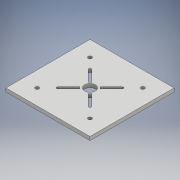
# Autodesk Inventor part: Base Robot
Saved by Autodesk Inventor 2017 (Build 210142000, 142)
## iProperties
Created: 2021-03-08
Part Number: Base Robot
Material: Generic
Document SubType Name: Modeling
Designer: Lenovo Y900
Density: 1 g/cm^3
Appearance: Default
Author: Lenovo Y900
Autodesk Inventor part; units mm, degrees
ref_plane "YZ Plane" through (0, 0, 0) normal (1, 0, 0) x (0, 1, 0)
ref_plane "XZ Plane" through (0, 0, 0) normal (0, 1, 0) x (-1, 0, 0)
ref_plane "XY Plane" through (0, 0, 0) normal (0, 0, 1) x (1, 0, 0)
sketch "Sketch1" plane through (0, 0, 0) normal (0, 0, 1) x (1, 0, 0)
  circle A0 centre (-22, 22) radius 1.5
  circle A1 centre (22, 22) radius 1.5
  circle A2 centre (22, -22) radius 1.5
  circle A3 centre (-22, -22) radius 1.5
  circle A4 centre (0, 0) radius 4.5
  line L0 (14.8492, 13.435) -> (-14.8492, -13.435) construction
  line L1 (13.435, -14.8492) -> (-13.435, 14.8492) construction
  line L2 (-14.8492, 13.435) -> (14.8492, -13.435) construction
  line L3 (-12.7279, 14.1421) -> (-3.4762, 4.8904) construction
  line L4 (-4.8904, 3.4762) -> (-14.1421, 12.7279)
  line L5 (-4.8904, -3.4762) -> (-14.1421, -12.7279)
  line L6 (-12.7279, -14.1421) -> (-3.4762, -4.8904)
  line L7 (12.7279, -14.1421) -> (3.4762, -4.8904)
  line L8 (-0.6718, -0.7425) -> (-0.7425, -0.6718)
  line L9 (0.6718, 0.7425) -> (0.7071, 0.7071)
  line L10 (4.8904, -3.4762) -> (14.1421, -12.7279)
  line L11 (0.6718, -0.7425) -> (0.7425, -0.6718)
  line L12 (4.8904, 3.4762) -> (14.1421, 12.7279)
  line L13 (12.7279, 14.1421) -> (3.4762, 4.8904)
  line L14 (-0.6718, 0.7425) -> (-0.7425, 0.6718)
  arc A5 (-12.7279, 14.1421) -> (-14.1421, 12.7279) centre (-13.435, 13.435) ccw
  arc A6 (14.1421, 12.7279) -> (12.7279, 14.1421) centre (13.435, 13.435) ccw
  arc A7 (-14.1421, -12.7279) -> (-12.7279, -14.1421) centre (-13.435, -13.435) ccw
  arc A8 (12.7279, -14.1421) -> (14.1421, -12.7279) centre (13.435, -13.435) ccw
  line L15 (-20.9393, -20.9393) -> (-22, -22)
  line L16 (-22, 22) -> (-20.9393, 20.9393)
  line L17 (22, 22) -> (20.9393, 20.9393)
  line L18 (20.9393, -20.9393) -> (22, -22)
  line L19 (-13.435, -14.8492) -> (4.0255, 4.4492) construction
  line L20 (12.9433, 14.3058) -> (13.435, 14.8492) construction
  line L21 (-12.7279, 14.1421) -> (-3.4762, 4.8904)
  arc A9 (-3.4762, 4.8904) -> (-4.8904, 3.4762) centre (0, 0) ccw
  arc A10 (-4.8904, -3.4762) -> (-3.4762, -4.8904) centre (0, 0) ccw
  arc A11 (3.4762, -4.8904) -> (4.8904, -3.4762) centre (0, 0) ccw
  arc A12 (4.8904, 3.4762) -> (3.4762, 4.8904) centre (0, 0) ccw
  line L22 (-35, -35) -> (35, -35)
  line L23 (35, -35) -> (35, 35)
  line L24 (35, 35) -> (-35, 35)
  line L25 (-35, 35) -> (-35, -35)
  line L26 (-35, -35) -> (35, 35) construction
  line L27 (35, -35) -> (-35, 35) construction
  dimension "d12" = 3
  dimension "d13" = 3
  dimension "d14" = 3
  dimension "d15" = 3
  dimension "d55" = 70
  dimension "d56" = 70
  constraints: 56 end point, 20 parallel, 18 point on circle, 9 centre point, 8 point on line, 5 midpoint, 2 coincident, 1 collinear, 1 horizontal, 1 perpendicular, 1 tangent, 12 other
  measures "d55" distance of L24.end L23.end
  measures "d56" distance of L23.end L22.end
extrude "Extrusion4" add sketch "Sketch1" along normal blind 3
body "Solid4"
